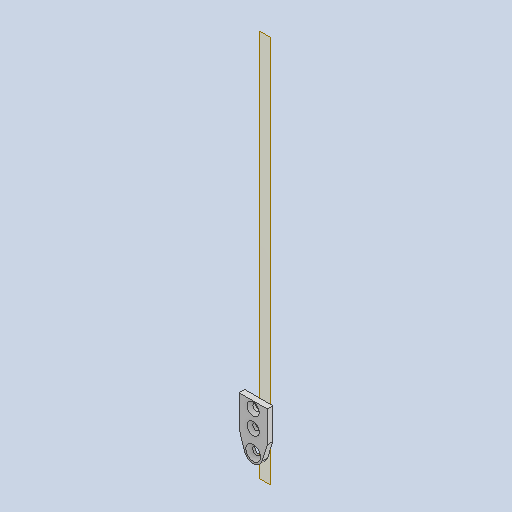
# Autodesk Inventor part: belt_tentioner_plane
Saved by Autodesk Inventor 2024 (Build 280153000, 153)
## iProperties
Created: 2026-02-05
Part Number: belt_tentioner_plane
Material: Generic
Document SubType Name: Modeling
Designer: SEMEN
Density: 1 g/cm^3
Appearance: Default
Author: SEMEN
Autodesk Inventor part; units mm, degrees
ref_plane "YZ Plane" through (0, 0, 0) normal (1, 0, 0) x (0, 1, 0)
ref_plane "XZ Plane" through (0, 0, 0) normal (0, 1, 0) x (-1, 0, 0)
ref_plane "XY Plane" through (0, 0, 0) normal (0, 0, 1) x (1, 0, 0)
ref_plane "Work Plane1" through (-2.1234, -14.9845, 0) normal (0, 0, 1) x (1, 0, 0)
sketch "Sketch1" plane through (-2.1234, -14.9845, 0) normal (0, 0, 1) x (1, 0, 0)
  line L0 (-10.8766, 764.9845) -> (-3.8766, 764.9845) projected
  line L1 (-3.8766, 764.9845) -> (-3.8766, 1014.9845) projected
  line L2 (-10.8766, 1014.9845) -> (-3.8766, 1014.9845) projected
  line L3 (-10.8766, 764.9845) -> (-10.8766, 1014.9845) projected
  line L4 (2.1234, 764.9845) -> (9.1234, 764.9845) projected
  line L5 (9.1234, 764.9845) -> (9.1234, 1014.9845) projected
  line L6 (2.1234, 1014.9845) -> (9.1234, 1014.9845) projected
  line L7 (2.1234, 764.9845) -> (2.1234, 1014.9845) projected
  circle A0 centre (-0.8766, 754.9845) radius 2.5 projected
  line L8 (-0.8766, 754.9845) -> (-0.8766, 786.7892) construction
  line L9 (-10.8766, 764.9845) -> (-7.0711, 753.0151)
  line L10 (5.3178, 753.0151) -> (9.1234, 764.9845)
  circle A1 centre (-0.8766, 754.9845) radius 6.5
  line L11 (-10.8766, 764.9845) -> (-10.8766, 786.9845)
  line L12 (-10.8766, 786.9845) -> (9.1234, 786.9845)
  line L13 (9.1234, 764.9845) -> (9.1234, 786.9845)
  point P0 (2.1234, 14.9845)
  point P1 (-0.8766, 769.9845)
  point P2 (-0.8766, 781.9845)
  dimension "d0" = 5
  dimension "d1" = 12
  dimension "d2" = 4
  dimension "d3" = 5
  constraints: 12 end point, 4 point on line, 2 point on circle, 2 tangent, 1 centre point, 1 collinear, 1 perpendicular, 1 vertical
  measures "d0" distance from line of L4 point (-0.877, 769.985)
  measures "d1" distance of point (-0.877, 769.985) point (-0.877, 781.985)
  measures "d2" radial gap between concentric circles of A0 A1
  measures "d3" distance from line of L12 point (-0.877, 781.985)
extrude "Extrusion1" add sketch "Sketch1" along normal blind 4 contours L3 L12 L1 L0 | L0 L1 L12 L7 L4 L10 A1 L9 | A1 | L12 L5 L4 L7 | A0
sketch "Sketch2" plane through (-2.1234, -14.9845, 4) normal (0, 0, 1) x (1, 0, 0)
  point P0 (2.1234, 14.9845)
  point P1 (-0.8766, 769.9845)
  point P2 (-0.8766, 781.9845)
  point P3 (-0.8766, 754.9845)
hole "Hole1" at (-3, 755, 4) at (-3, 767, 4) direction (0, 0, -1) diameter 4.5 end through all countersink diameter 8.6 countersink angle 90 clearance for "Countersunk Head GOST 12876-67" size "M4" standard "GOST"
hole "Hole2" at (-3, 740, 4) direction (0, 0, -1) diameter 5.5 end through all countersink diameter 10.4 countersink angle 90 clearance for "Countersunk Head GOST 12876-67" size "M5" standard "GOST"
body "Solid1"
